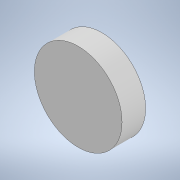
# Autodesk Inventor part: soporte base pila
Saved by Autodesk Inventor 2021 (Build 250183000, 183)
## iProperties
Created: 2020-11-18
Part Number: soporte base pila
Material: Generic
Document SubType Name: Modeling
Designer: Miguel
Density: 1 g/cm^3
Appearance: Default
Author: Miguel
Autodesk Inventor part; units mm, degrees
ref_plane "YZ Plane" through (0, 0, 0) normal (1, 0, 0) x (0, 1, 0)
ref_plane "XZ Plane" through (0, 0, 0) normal (0, 1, 0) x (-1, 0, 0)
ref_plane "XY Plane" through (0, 0, 0) normal (0, 0, 1) x (1, 0, 0)
sketch "Sketch1" plane through (0, 0, 0) normal (0, 0, 1) x (1, 0, 0)
  circle A0 centre (0, 0) radius 27.9
  line L0 (-24, 12.5) -> (24, 12.5)
  line L1 (24, 12.5) -> (24, -12.5)
  line L2 (24, -12.5) -> (-24, -12.5)
  line L3 (-24, -12.5) -> (-24, 12.5)
  dimension "d0" = 55.8
  dimension "d1" = 48
  dimension "d2" = 24
  dimension "d3" = 25
  dimension "d4" = 12.5
  constraints: 8 end point, 2 parallel, 1 centre point, 1 coincident, 1 horizontal, 1 perpendicular
  measures "d0" diameter of A0
  measures "d1" distance between parallel lines of L1 L3
  measures "d2" distance from line of point (0, 0) L3
  measures "d3" distance between parallel lines of L2 L0
  measures "d4" distance from line of point (0, 0) L0
extrude "Extrusion1" add sketch "Sketch1" along normal mid plane 15
sketch "Sketch2" plane through (0, 0, 7.5) normal (0, 0, 1) x (1, 0, 0)
  circle A0 centre (0, 0) radius 27.9
  dimension "d10" = 55.8
  constraints: 1 centre point, 1 coincident
  measures "d10" diameter of A0
extrude "Extrusion2" add sketch "Sketch2" against normal blind 5
fillet "Fillet1" radius 1 4 edges at (-24, 0, -7.5) (0, 12.5, -7.5) (0, -12.5, -7.5) (24, 0, -7.5)
equation "\"d2\" = 0.5 * d1"
equation "\"d4\" = 0.5 * d3"
body "Solid1"
